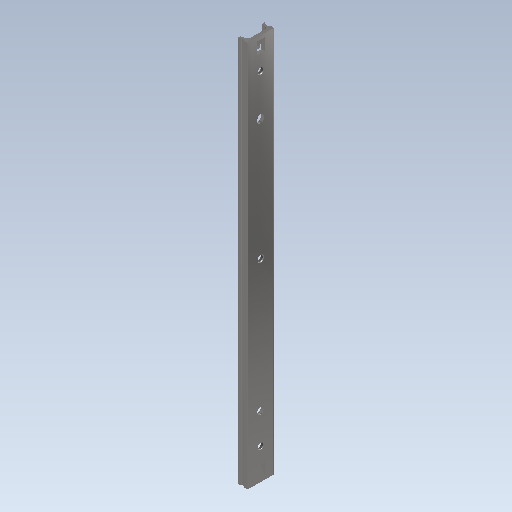
# Autodesk Inventor part: SSRC215_ir
Saved by Autodesk Inventor 2021.2 (Build 252289000, 289)
## iProperties
Part Number: SSRC215_ir
Material: ステンレス鋼
Catalog Web Link: www.cadenas.de
Description: SSRC2_inner_rail-Slide Rails - Load Rating: 137N ~ 177N/2 pcs - Light Load / Compact - Stainless Steel - Tow-Step
Vendor: MISUMI
Document SubType Name: Modeling
Designer: partserver
Manufacturer: MISUMI
Mass: 20.016 g
Surface Area: 47.815 cm^2
Volume: 2.502 cm^3
Density: 8 g/cm^3
Appearance: 半つや出し
Category: PARTsolutions
Company: MISUMI
PSOL_IDENT_0: {$CADENAS_DATA\23d-libs\misumi\metric\07_slide_rails\ssrc2\ssrc2_inner_rail.prj},167 {VTYP=3D},{NB=S
PSOL_IDENT_1: SRC215_ir},{LINA=SSRC215},{NN=SSRC2_inner_rail},{DATE=30.03.2018 01:39:53},{GEOMDATE=30.06.2015 02:0
PSOL_IDENT_2: 1:01},{VERSION=},{LINEID=30},{WBVAR=},{WBNUMERIC=}  {NB=SSRC215_ir},{LINA=SSRC215},{KT=DUMMY},{PN=SS
PSOL_IDENT_3: RC215},{TYPE=SSRC2},{NO=15},{L=150},{S=94.5},{A=63},{B=126},{C=63},{D=126},{E=102},{F=98}
NB: SSRC215_ir
NN: SSRC2_inner_rail
NT: Slide Rails - Load Rating: 137N ~ 177N/2 pcs - Light Load / Compact - Stainless Steel - Tow-Step
NBSYN: $PN._ir
LINA: SSRC215
CATALOG: Misumi
PN: SSRC215
NO: 15
L: 150
S: 94.5
A: 63
B: 126
C: 63
D: 126
E: 102
F: 98
SUPPLIER: MISUMI
ARTICLENO: SSRC215_ir
BOMINFO: SSRC215
CREATOR: CADENAS GmbH
Title: SSRC215
Author: Cadenas PARTsolutions
Comments: Slide Rails - Load Rating: 137N ~ 177N/2 pcs - Light Load / Compact - Stainless Steel - Tow-Step
Autodesk Inventor part; units mm, degrees
sketch "_____1" plane through (0, 0, 0) normal (0, 0, 1) x (1, 0, 0)
  line L0 (-2.35, 4.9) -> (-2.35, -4.9)
  arc A0 (-2.35, -4.9) -> (-2.15, -5.1) centre (-2.15, -4.9) ccw
  line L1 (-2.15, -5.1) -> (-1.1124, -5.1)
  arc A1 (-1.1124, -5.1) -> (-0.9535, -5.0214) centre (-1.1124, -4.9) ccw
  arc A2 (0.9535, -5.0214) -> (-0.9535, -5.0214) centre (0, -5.75) ccw
  arc A3 (0.9535, -5.0214) -> (1.1124, -5.1) centre (1.1124, -4.9) ccw
  line L2 (1.1124, -5.1) -> (1.2, -5.1)
  arc A4 (1.2, -5.1) -> (1.3, -5) centre (1.2, -5) ccw
  line L3 (1.3, -5) -> (1.3, -4.3536)
  arc A5 (1.3, -4.3536) -> (1.1517, -4.1603) centre (1.1, -4.3536) ccw
  line L4 (1.1517, -4.1603) -> (-0.4083, -3.7433)
  arc A6 (-1.15, -2.7772) -> (-0.4083, -3.7433) centre (-0.15, -2.7772) ccw
  line L5 (-1.15, -2.7772) -> (-1.15, 2.7772)
  arc A7 (-0.4083, 3.7433) -> (-1.15, 2.7772) centre (-0.15, 2.7772) ccw
  line L6 (-0.4083, 3.7433) -> (1.1517, 4.1603)
  arc A8 (1.1517, 4.1603) -> (1.3, 4.3536) centre (1.1, 4.3536) ccw
  line L7 (1.3, 4.3536) -> (1.3, 5)
  arc A9 (1.3, 5) -> (1.2, 5.1) centre (1.2, 5) ccw
  line L8 (1.2, 5.1) -> (1.1124, 5.1)
  arc A10 (1.1124, 5.1) -> (0.9535, 5.0214) centre (1.1124, 4.9) ccw
  arc A11 (-0.9535, 5.0214) -> (0.9535, 5.0214) centre (0, 5.75) ccw
  arc A12 (-0.9535, 5.0214) -> (-1.1124, 5.1) centre (-1.1124, 4.9) ccw
  line L9 (-1.1124, 5.1) -> (-2.15, 5.1)
  arc A13 (-2.15, 5.1) -> (-2.35, 4.9) centre (-2.15, 4.9) ccw
  constraints: 28 point on circle, 20 end point, 14 centre point
extrude "Extrusion1" add sketch "_____1" against normal blind 150
sketch "_____2" plane through (-2.35, 0, 0) normal (1, 0, 0) x (0, 0, -1)
  line L0 (1.4, 1.5) -> (1.4, -1.5)
  line L1 (1.4, -1.5) -> (5.9, -1.5)
  line L2 (5.9, -1.5) -> (5.9, 1.5)
  line L3 (5.9, 1.5) -> (1.4, 1.5)
  constraints: 8 end point
extrude "Extrusion2" cut sketch "_____2" along normal blind 1.2
sketch "_____3" plane through (-2.35, 0, 0) normal (1, 0, 0) x (0, 0, -1)
  line L0 (144.1, 1.5) -> (144.1, -1.5)
  line L1 (144.1, -1.5) -> (148.6, -1.5)
  line L2 (148.6, -1.5) -> (148.6, 1.5)
  line L3 (148.6, 1.5) -> (144.1, 1.5)
  constraints: 8 end point
extrude "Extrusion3" cut sketch "_____3" along normal blind 1.2
sketch "_____4" plane through (0, 0, 0) normal (0, 1, 0) x (1, 0, 0)
  line L0 (-2.35, 1.4) -> (-1.15, 1.4)
  line L1 (-1.15, 1.4) -> (0.65, 4.9)
  line L2 (0.65, 4.9) -> (0.65, 5.9)
  line L3 (0.65, 5.9) -> (-0.55, 5.9)
  line L4 (-0.55, 5.9) -> (-0.55, 4.9)
  line L5 (-0.55, 4.9) -> (-2.35, 1.4)
  constraints: 12 end point
extrude "Extrusion4" add sketch "_____4" along normal mid plane 3
sketch "_____5" plane through (0, 0, 0) normal (0, 1, 0) x (1, 0, 0)
  line L0 (-2.35, 148.6) -> (-0.55, 145.1)
  line L1 (-0.55, 145.1) -> (-0.55, 144.1)
  line L2 (-0.55, 144.1) -> (0.65, 144.1)
  line L3 (0.65, 144.1) -> (0.65, 145.1)
  line L4 (0.65, 145.1) -> (-1.15, 148.6)
  line L5 (-1.15, 148.6) -> (-2.35, 148.6)
  constraints: 12 end point
extrude "Extrusion5" add sketch "_____5" along normal mid plane 3
sketch "_____6" plane through (0, 0, 0) normal (0, 1, 0) x (1, 0, 0)
  line L0 (-1.15, 12) -> (-2.35, 12)
  line L1 (-2.35, 12) -> (-2.35, 13.3)
  line L2 (-2.35, 13.3) -> (-2.1065, 13.0565)
  line L3 (-2.1065, 13.0565) -> (-1.3935, 13.0565)
  line L4 (-1.3935, 13.0565) -> (-1.15, 13.3)
  line L5 (-1.15, 13.3) -> (-1.15, 12)
  line L6 (-1.15, 12) -> (-2.35, 12)
  constraints: 14 end point
revolve "Revolution1" cut sketch "_____6" angle 360 about axis through (-1.15, 0, -12) along (1, 0, 0)
thread "Thread1" size "M2.6x0.45" class "6H" standard "ISO Metric profile" full length
pattern_linear "Rectangular Pattern1" count 2 spacing 126 along (0, 0, -1) of "Revolution1"
sketch "_____10" plane through (0, 0, 0) normal (0, 1, 0) x (1, 0, 0)
  line L0 (-1.15, 75) -> (-2.35, 75)
  line L1 (-2.35, 75) -> (-2.35, 76.3)
  line L2 (-2.35, 76.3) -> (-2.1065, 76.0565)
  line L3 (-2.1065, 76.0565) -> (-1.3935, 76.0565)
  line L4 (-1.3935, 76.0565) -> (-1.15, 76.3)
  line L5 (-1.15, 76.3) -> (-1.15, 75)
  line L6 (-1.15, 75) -> (-2.35, 75)
  constraints: 14 end point
revolve "Revolution2" cut sketch "_____10" angle 360 about axis through (-1.15, 0, -75) along (1, 0, 0)
thread "Thread2" size "M2.6x0.45" class "6H" standard "ISO Metric profile" full length
sketch "Sketch8" plane through (-1.15, -2.7772, 0) normal (1, 0, 0) x (0, 0, -1)
  point P0 (24, 2.7772)
hole "Hole1" at (-1.15, 0, -24) direction (-1, 0, 0) diameter 2.8 depth 1.2
sketch "_____8" plane through (-1.15, 0, 0) normal (1, 0, 0) x (0, 0, -1)
  arc A0 (121.8, 1.4) -> (121.8, -1.4) centre (121.8, 0) ccw
  line L0 (121.8, -1.4) -> (122.2, -1.4)
  arc A1 (122.2, -1.4) -> (122.2, 1.4) centre (122.2, 0) ccw
  line L1 (122.2, 1.4) -> (121.8, 1.4)
  constraints: 4 end point, 4 point on circle, 2 centre point
extrude "Extrusion6" cut sketch "_____8" against normal blind 1.2
ref_plane "to_retainer_XY" through (0, 0, -150) normal (0, 0, -1) x (1, 0, 0)
ref_plane "to_retainer_YZ" through (0, 0, -150) normal (1, 0, 0) x (0, -1, 0)
ref_plane "to_retainer_ZX" through (0, 0, -150) normal (0, -1, 0) x (0, 0, -1)
body "Solid1"
